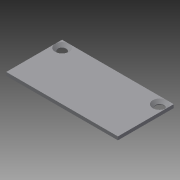
# Autodesk Inventor part: Back
Saved by Autodesk Inventor 2015 (Build 190159000, 159)
## iProperties
Created: 2018-04-13
Part Number: Back
Material: Generic
Document SubType Name: Modeling
Designer: Toby
Density: 1 g/cm^3
Appearance: Default
Author: Toby
Autodesk Inventor part; units mm, degrees
ref_plane "YZ Plane" through (0, 0, 0) normal (1, 0, 0) x (0, 1, 0)
ref_plane "XZ Plane" through (0, 0, 0) normal (0, 1, 0) x (-1, 0, 0)
ref_plane "XY Plane" through (0, 0, 0) normal (0, 0, 1) x (1, 0, 0)
sketch "Sketch1" plane through (0, 0, 0) normal (0, 0, 1) x (1, 0, 0)
  line L0 (-30.5445, 14.7145) -> (9.4555, 14.7145)
  line L1 (9.4555, 14.7145) -> (9.4555, -5.2855)
  line L2 (9.4555, -5.2855) -> (-30.5445, -5.2855)
  line L3 (-30.5445, -5.2855) -> (-30.5445, 14.7145)
  point P0 (0, 0)
  dimension "d0" = 40
  dimension "d1" = 20
  constraints: 8 end point, 2 parallel, 1 horizontal, 1 perpendicular
  measures "d0" distance of L0.start L0.end
  measures "d1" distance of L2.end L0.start
extrude "Extrusion1" add sketch "Sketch1" along normal blind 1.2
sketch "Sketch2" plane through (0, 0, 1.2) normal (0, 0, 1) x (1, 0, 0)
  line L0 (-30.5445, 14.7145) -> (9.4555, 14.7145) projected
  line L1 (-30.5445, -5.2855) -> (-30.5445, 14.7145) projected
  line L2 (9.4555, 14.7145) -> (9.4555, -5.2855) projected
  point P0 (0, 0)
  point P1 (-28.0445, 12.2145)
  point P2 (6.9555, 12.2145)
  dimension "d4" = 2.5
  dimension "d5" = 2.5
  dimension "d6" = 2.5
  dimension "d7" = 2.5
  measures "d4" distance from line of L0 point (-28.044, 12.214)
  measures "d5" distance from line of L1 point (-28.044, 12.214)
  measures "d6" distance from line of L0 point (6.956, 12.214)
  measures "d7" distance from line of L2 point (6.956, 12.214)
hole "Hole1" at (-28.0445, 12.2145, 1.2) at (6.9555, 12.2145, 1.2) direction (0, 0, -1) diameter 3 depth 8 tip angle 118 countersink diameter 5 countersink angle 90
body "Solid1"
